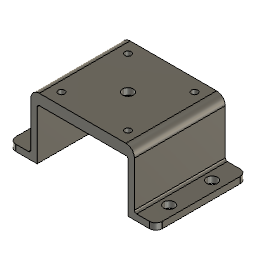
nema_extrude (Autodesk Fusion 360 design; units mm, degrees)
Autodesk Fusion 360 part; units mm, degrees
sketch "Sketch1" plane through (0, 0, 0) normal (0, 0, 1) x (1, 0, 0)
  line L0 (-21.15, 21.15) -> (21.15, 21.15)
  line L1 (21.15, 21.15) -> (21.15, -21.15)
  line L2 (21.15, -21.15) -> (-21.15, -21.15)
  line L3 (-21.15, -21.15) -> (-21.15, 21.15)
  line L4 (-21.15, 21.15) -> (21.15, -21.15) construction
  line L5 (21.15, 21.15) -> (-21.15, -21.15) construction
  line L6 (-15.5, 15.5) -> (15.5, 15.5) construction
  line L7 (15.5, 15.5) -> (15.5, -15.5) construction
  line L8 (15.5, -15.5) -> (-15.5, -15.5) construction
  line L9 (-15.5, -15.5) -> (-15.5, 15.5) construction
  line L10 (-15.5, 15.5) -> (15.5, -15.5) construction
  line L11 (15.5, 15.5) -> (-15.5, -15.5) construction
  circle A0 centre (-15.5, 15.5) radius 1.5
  circle A1 centre (-15.5, -15.5) radius 1.5
  circle A2 centre (15.5, -15.5) radius 1.5
  circle A3 centre (15.5, 15.5) radius 1.5
  circle A4 centre (0, 0) radius 2.5
  circle A5 centre (0, 0) radius 11
  line L12 (-21.15, -21.15) -> (-24.15, -21.15)
  line L13 (-24.15, -21.15) -> (-24.15, 21.15)
  line L14 (-24.15, 21.15) -> (-21.15, 21.15)
  line L15 (-21.15, 21.15) -> (-21.15, -21.15)
  line L16 (21.15, -21.15) -> (24.15, -21.15)
  line L17 (24.15, -21.15) -> (24.15, 21.15)
  line L18 (24.15, 21.15) -> (21.15, 21.15)
  line L19 (21.15, 21.15) -> (21.15, -21.15)
  dimension "d1" = 42.3
  dimension "d2" = 42.3
  dimension "d5" = 31
  dimension "d6" = 31
  dimension "d8" = 3
  dimension "d10" = 360
  dimension "d12" = 5
  dimension "d14" = 22
  dimension "d17" = 3
  dimension "d18" = 42.3
  dimension "d19" = 3
  dimension "d20" = 42.3
  constraint horizontal L0
  constraint perpendicular L0 L1
  constraint parallel L0 L2
  constraint parallel L1 L3
  constraint coincident L4 A4.centre
  constraint coincident L5 A4.centre
  constraint coincident A4.centre A5.centre
  constraint horizontal L6
  constraint perpendicular L6 L7
  constraint parallel L6 L8
  constraint parallel L7 L9
  constraint coincident L10 A4.centre
  constraint coincident L11 A4.centre
  constraint coincident L6.start L9.end
  constraint concentric A4 A5
  constraint horizontal L12
  constraint vertical L13
  constraint horizontal L14
  constraint vertical L15
  constraint horizontal L16
  constraint vertical L17
  constraint horizontal L18
  constraint vertical L19
  measures "d1" distance of L1.end L2.end
  measures "d2" distance of L0.end L1.end
  measures "d5" distance of L7.end L8.end
  measures "d6" distance of L6.end L7.end
  measures "d8" diameter of A0
  measures "d12" diameter of A4
  measures "d14" diameter of A5
  measures "d17" distance of L2.end L12.end
  measures "d18" distance of L2.end L0.start
  measures "d19" distance of L1.end L16.end
  measures "d20" distance of L1.end L0.end
extrude "Extrude1" add sketch "Sketch1" along normal blind 5 contours L0 L1 L2 L3 L15 L19 | L3 L12 L13 L14 L15 | L1 L16 L17 L18 L19 | A5
extrude "Extrude2" add sketch "Sketch1" against normal blind 24 contours L3 L12 L13 L14 L15 | L1 L16 L17 L18 L19
extrude "Extrude3" cut sketch "Sketch1" along normal blind 2 contours A5
sketch "Sketch2" plane through (24.15, 0, 0) normal (1, 0, 0) x (0, 1, 0)
  line L0 (-21.15, 5) -> (-21.15, -24)
  line L1 (-21.15, -24) -> (21.15, -24)
  line L2 (21.15, -24) -> (21.15, 5)
  line L3 (-21.15, -24) -> (21.15, -24)
  line L4 (21.15, -24) -> (21.15, -21)
  line L5 (21.15, -21) -> (-21.15, -21)
  line L6 (-21.15, -21) -> (-21.15, -24)
  line L7 (21.15, 5) -> (-21.15, 5)
  dimension "d28" = 42.3
  dimension "d29" = 3
  constraint horizontal L3
  constraint vertical L4
  constraint horizontal L5
  constraint vertical L6
  constraint coincident L0.end L1.start
  measures "d28" distance of L0.end L1.end
  measures "d29" distance of L0.end L5.end
extrude "Extrude4" add sketch "Sketch2" along normal blind 10 contours L0 L1 L2 L3 L4 L5 L6
sketch "Sketch3" plane through (-24.15, 0, 0) normal (-1, 0, 0) x (0, -1, 0)
  line L0 (21.15, -24) -> (21.15, 5)
  line L1 (21.15, 5) -> (-21.15, 5)
  line L2 (-21.15, 5) -> (-21.15, -24)
  line L3 (-21.15, -24) -> (21.15, -24)
  line L4 (-21.15, -24) -> (21.15, -24)
  line L5 (21.15, -24) -> (21.15, -21)
  line L6 (21.15, -21) -> (-21.15, -21)
  line L7 (-21.15, -21) -> (-21.15, -24)
  dimension "d32" = 42.3
  dimension "d33" = 3
  constraint horizontal L4
  constraint vertical L5
  constraint horizontal L6
  constraint vertical L7
  constraint coincident L2.end L3.start
  measures "d32" distance of L2.end L0.start
  measures "d33" distance of L2.end L6.end
extrude "Extrude5" add sketch "Sketch3" along normal blind 10 contours L0 L2 L3 L4 L5 L6 L7
sketch "Sketch4" plane through (0, 0, -21) normal (0, 0, 1) x (-1, 0, 0)
  line L0 (24.15, 21.15) -> (24.15, -21.15)
  line L1 (24.15, -21.15) -> (34.15, -21.15)
  line L2 (34.15, -21.15) -> (34.15, 21.15)
  line L3 (34.15, 21.15) -> (24.15, 21.15)
  line L4 (24.15, 0) -> (34.15, 0) construction
  line L5 (29.15, 0) -> (29.15, 10) construction
  circle A0 centre (29.15, 10) radius 2.5
  circle A1 centre (29.15, -10) radius 2.5
  dimension "d36" = 10
  dimension "d38" = 5
  constraint midpoint L0 L4.start
  constraint midpoint L2 L4.end
  constraint midpoint L4 L5.start
  constraint perpendicular L4 L5
  constraint coincident L5.end A0.centre
  constraint symmetric L4 A0 A1
  measures "d36" distance of L5.start L5.end
  measures "d38" diameter of A0
extrude "Extrude6" cut sketch "Sketch4" against normal blind 3 contours A0 | A1
sketch "Sketch5" plane through (0, 0, -21) normal (0, 0, 1) x (-1, 0, 0)
  line L0 (-24.15, -21.15) -> (-24.15, 21.15)
  line L1 (-24.15, 21.15) -> (-34.15, 21.15)
  line L2 (-34.15, 21.15) -> (-34.15, -21.15)
  line L3 (-34.15, -21.15) -> (-24.15, -21.15)
  line L4 (-34.15, 0) -> (-24.15, 0) construction
  line L5 (-29.15, 0) -> (-29.15, 10) construction
  circle A0 centre (-29.15, 10) radius 2.5
  circle A1 centre (-29.15, -10) radius 2.5
  dimension "d41" = 10
  dimension "d42" = 5
  constraint midpoint L2 L4.start
  constraint midpoint L0 L4.end
  constraint midpoint L4 L5.start
  constraint perpendicular L4 L5
  constraint coincident L5.end A0.centre
  constraint symmetric L4 A0 A1
  measures "d41" distance of L5.start L5.end
  measures "d42" diameter of A0
extrude "Extrude7" cut sketch "Sketch5" against normal blind 3 contours A0 | A1
fillet "Fillet1" radius 3 4 edges at (34.15, 21.15, -22.5) (34.15, -21.15, -22.5) (-34.15, 21.15, -22.5) (-34.15, -21.15, -22.5)
fillet "Fillet2" radius 4 2 edges at (24.15, 0, 5) (-24.15, 0, 5)
fillet "Fillet3" radius 1 2 edges at (21.15, 0, 0) (-21.15, 0, 0)
fillet "Fillet3" radius 1 2 edges at (24.15, 0, -21) (-24.15, 0, -21)
equation "d1 = nema_l"
equation "d2 = nema_l"
equation "nema_l = 42.3 mm"
equation "nema_spacing = 31 mm"
equation "d5 = nema_spacing"
equation "d6 = nema_spacing"
equation "nema_hole = 3 mm"
equation "d8 = nema_hole"
equation "nema_shaft = 5 mm"
equation "d12 = nema_shaft"
equation "nema_disc = 22 mm"
equation "d14 = nema_disc"
equation "thick_vert = 3 mm"
equation "thick_hori = 3 mm"
equation "d17 = thick_vert"
equation "d18 = nema_l"
equation "d19 = thick_vert"
equation "d20 = nema_l"
equation "d21 = 2 mm + thick_hori"
equation "height = 24 mm"
equation "d24 = -( height )"
equation "d28 = nema_l"
equation "d29 = thick_hori"
equation "d32 = nema_l"
equation "d33 = thick_hori"
equation "alu_hole = 5 mm"
equation "d38 = alu_hole"
equation "d39 = -thick_hori"
equation "d42 = alu_hole"
equation "d43 = -thick_hori"
